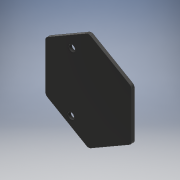
# Autodesk Inventor part: Kicker PCB
Saved by Autodesk Inventor 2017 (Build 210142000, 142)
## iProperties
Created: 2017-03-21
Part Number: Kicker PCB
Material: Generic
Document SubType Name: Modeling
Designer: yella
Density: 1 g/cm^3
Appearance: Smooth - Black
Author: yella
Autodesk Inventor part; units mm, degrees
ref_plane "YZ Plane" through (0, 0, 0) normal (1, 0, 0) x (0, 1, 0)
ref_plane "XZ Plane" through (0, 0, 0) normal (0, 1, 0) x (-1, 0, 0)
ref_plane "XY Plane" through (0, 0, 0) normal (0, 0, 1) x (1, 0, 0)
sketch "Sketch1" plane through (0, 0, 0) normal (0, 1, 0) x (-1, 0, 0)
  line L0 (55.4027, 26.2487) -> (74.9027, 14.9904)
  line L1 (75.9027, 13.2583) -> (75.9027, -9.2583)
  line L2 (74.9027, -10.9904) -> (55.4027, -22.2487)
  line L3 (53.4027, -22.2487) -> (33.9027, -10.9904)
  line L4 (32.9027, -9.2583) -> (32.9027, 13.2583)
  line L5 (33.9027, 14.9904) -> (53.4027, 26.2487)
  arc A0 (33.9027, 14.9904) -> (32.9027, 13.2583) centre (34.9027, 13.2583) ccw
  arc A1 (32.9027, -9.2583) -> (33.9027, -10.9904) centre (34.9027, -9.2583) ccw
  arc A2 (53.4027, -22.2487) -> (55.4027, -22.2487) centre (54.4027, -20.5167) ccw
  arc A3 (74.9027, -10.9904) -> (75.9027, -9.2583) centre (73.9027, -9.2583) ccw
  arc A4 (75.9027, 13.2583) -> (74.9027, 14.9904) centre (73.9027, 13.2583) ccw
  arc A5 (55.4027, 26.2487) -> (53.4027, 26.2487) centre (54.4027, 24.5167) ccw
  circle A6 centre (63.1527, -13.1554) radius 1.6
  circle A7 centre (62.6527, 16.2894) radius 1.6
  point P0 (0, 0)
  point P1 (54.4027, 26.8261)
  point P2 (75.9027, 14.413)
  point P3 (75.9027, -10.413)
  point P4 (54.4027, -22.8261)
  point P5 (32.9027, -10.413)
  point P6 (32.9027, 14.413)
  dimension "d0" = 3.2
  dimension "d1" = 3.2
  constraints: 12 end point, 12 point on circle, 12 point on line, 12 tangent, 8 centre point, 5 equal radius
  measures "d0" diameter of A6
  measures "d1" diameter of A7
extrude "Extrusion1" add sketch "Sketch1" along normal blind 1.4
body "Solid1"
